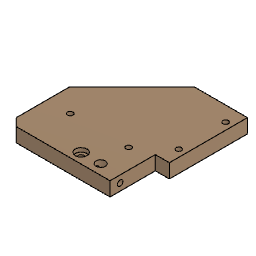
Brace BR (Autodesk Fusion 360 design; units mm, degrees)
Autodesk Fusion 360 part; units mm, degrees
sketch "Top" plane through (0, 0, 0) normal (0, 0, 1) x (1, 0, 0)
  line L0 (-18, 0) -> (-138, 0)
  line L1 (-148, 10) -> (-148, 78)
  line L2 (-68, 158) -> (0, 158)
  line L3 (0, 158) -> (0, 58)
  line L4 (-138, 0) -> (-148, 10)
  line L5 (-18, 0) -> (-18, 58)
  line L6 (-18, 58) -> (0, 58)
  line L7 (-9, 158) -> (-9, 58) construction
  circle A0 centre (-9, 79) radius 3.5
  circle A1 centre (-9, 139) radius 3.5
  line L8 (-18, 49) -> (-148, 49) construction
  circle A2 centre (-43, 49) radius 3.5
  circle A3 centre (-118, 49) radius 3.5
  circle A4 centre (-43, 13) radius 6
  circle A5 centre (-68, 13) radius 3.5
  circle A6 centre (-68, 13) radius 7.5
  line L9 (-148, 78) -> (-68, 158)
  dimension "d4" = 158
  dimension "d5" = 10
  dimension "d6" = 10
  dimension "d7" = 58
  dimension "d8" = 18
  dimension "d9" = 148
  dimension "d11" = 9
  dimension "d12" = 7
  dimension "d13" = 7
  dimension "d14" = 21
  dimension "d15" = 60
  dimension "d16" = 49
  dimension "d17" = 7
  dimension "d18" = 7
  dimension "d19" = 25
  dimension "d20" = 75
  dimension "d21" = 12
  dimension "d22" = 13
  dimension "d23" = 7
  dimension "d24" = 15
  dimension "d25" = 25
  dimension "d26" = 25
  dimension "d27" = 68
  dimension "d28" = 68
  constraint horizontal L0
  constraint vertical L1
  constraint horizontal L2
  constraint vertical L3
  constraint vertical L5
  constraint horizontal L6
  constraint coincident L2 L7.start
  constraint midpoint L6 L7.end
  constraint perpendicular L2 L7
  constraint coincident L7 A0.centre
  constraint coincident L7 A1.centre
  constraint coincident L5 L8.start
  constraint coincident L1 L8.end
  constraint perpendicular L1 L8
  constraint coincident L8 A2.centre
  constraint coincident L8 A3.centre
  constraint concentric A5 A6
  measures "d4" distance of origin L2.end
  measures "d5" vertical distance of L0.end L1.start
  measures "d6" horizontal distance of L0.end L1.start
  measures "d7" distance of origin L3.end
  measures "d8" distance of origin L0.start
  measures "d9" horizontal distance of origin L1.start
  measures "d11" distance of L3 L7
  measures "d12" diameter of A0
  measures "d13" diameter of A1
  measures "d14" distance of L6 A0.centre
  measures "d15" distance of A0.centre A1.centre
  measures "d16" distance of L0 L8
  measures "d17" diameter of A2
  measures "d18" diameter of A3
  measures "d19" distance of L5 A2.centre
  measures "d20" distance of A2.centre A3.centre
  measures "d21" diameter of A4
  measures "d22" distance of L0 A4.centre
  measures "d23" diameter of A5
  measures "d24" diameter of A6
  measures "d25" distance of A4.centre A5.centre
  measures "d26" distance of L5 A4.centre
  measures "d27" distance of L2.end L2.start
  measures "d28" distance of L1.start L1.end
extrude "Extrude1" add sketch "Top" along normal blind 13 contours A6
extrude "Extrude2" add sketch "Top" along normal blind 18 contours L0 L1 L2 L3 L4 L5 L6 L9
sketch "Side" plane through (-18, 0, 0) normal (1, 0, 0) x (0, 1, 0)
  line L0 (0, 0) -> (58, 0)
  line L1 (58, 0) -> (58, 18)
  line L2 (58, 18) -> (0, 18)
  line L3 (0, 18) -> (0, 0)
  line L4 (0, 0) -> (58, 0) construction
  line L5 (58, 0) -> (58, 18) construction
  line L6 (58, 18) -> (0, 18) construction
  line L7 (0, 18) -> (0, 0) construction
  line L8 (0, 9) -> (58, 9) construction
  circle A0 centre (13, 9) radius 3.5
  dimension "d33" = 7
  dimension "d34" = 13
  constraint horizontal L4
  constraint vertical L5
  constraint horizontal L6
  constraint vertical L7
  constraint coincident L1.end L2.start
  constraint coincident L0.start L3.end
  constraint midpoint L7 L8.start
  constraint midpoint L1 L8.end
  constraint coincident L8 A0.centre
  measures "d33" diameter of A0
  measures "d34" distance of L8.start A0.centre
extrude "Extrude3" cut sketch "Side" against normal blind 35 contours A0
named bodies: "Brace BR"
